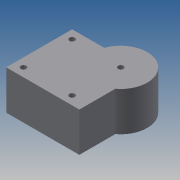
# Autodesk Inventor part: TITAN MOCKUP
Saved by Autodesk Inventor 2013 (Build 170138000, 138)
## iProperties
Created: 2017-04-01
Part Number: TITAN MOCKUP
Material: Generic
Document SubType Name: Modeling
Designer: employee
Density: 1 g/cm^3
Author: employee
Autodesk Inventor part; units mm, degrees
ref_plane "YZ Plane" through (0, 0, 0) normal (1, 0, 0) x (0, 1, 0)
ref_plane "XZ Plane" through (0, 0, 0) normal (0, 1, 0) x (-1, 0, 0)
ref_plane "XY Plane" through (0, 0, 0) normal (0, 0, 1) x (1, 0, 0)
sketch "Sketch1" plane through (0, 0, 0) normal (0, 0, 1) x (1, 0, 0)
  line L0 (-21, 21) -> (21, 21)
  line L1 (21, 21) -> (21, -21)
  line L2 (21, -21) -> (-21, -21)
  line L3 (-21, -21) -> (-21, 21)
  line L4 (15.5, 15.5) -> (-15.5, 15.5) construction
  line L5 (-15.5, 15.5) -> (-15.5, -15.5)
  line L6 (-15.5, -15.5) -> (15.5, -15.5) construction
  line L7 (15.5, -15.5) -> (15.5, 15.5)
  circle A0 centre (-15.5, 15.5) radius 1.75
  circle A1 centre (15.5, 15.5) radius 1.75
  circle A2 centre (-15.5, -15.5) radius 1.75
  circle A3 centre (15.5, -15.5) radius 1.75
  point P0 (0, 0)
  point P1 (0, 0)
  dimension "d0" = 42
  dimension "d1" = 5.5
  dimension "d2" = 3.5
  constraints: 16 end point, 5 coincident, 4 centre point, 3 equal radius, 1 horizontal, 12 other
  measures "d0" distance of L0.start L0.end
  measures "d1" distance from line of L0 L4.end
  measures "d2" diameter of A0
extrude "Extrusion1" add sketch "Sketch1" along normal blind 25
sketch "Sketch2" plane through (21, -21, 0) normal (1, 0, 0) x (0, 0, -1)
  line L0 (0, 42) -> (0, 0) projected
  line L1 (0, 42) -> (-25, 42) projected
  line L2 (-25, 0) -> (-25, 42) projected
  line L3 (0, 0) -> (-25, 0) projected
  point P0 (0, 21)
extrude "Extrusion2" add sketch "Sketch2" along normal blind 4.6
sketch "Sketch3" plane through (0, 0, 25) normal (0, 0, 1) x (1, 0, 0)
  circle A0 centre (15.5, 15.5) radius 1.75 projected
  line L0 (25.6, 21) -> (25.6, -21) projected
  circle A1 centre (15.5, 15.5) radius 16.9
  line L1 (25.6, 15.5) -> (32.4, 15.5)
  point P0 (0, 0)
  dimension "d7" = 16.9
  constraints: 2 end point, 2 horizontal alignment, 1 coincident, 1 perpendicular, 1 point on line, 2 other
  measures "d7" distance of L1.end point (15.5, 15.5)
extrude "Extrusion3" add sketch "Sketch3" against normal up to surface (25 mm away)
body "Solid1"
